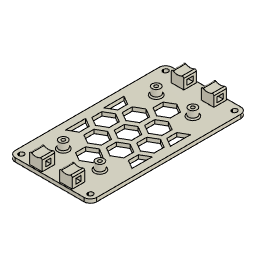
Lower Bay Tray - BIGTREETECH Relay 1.2 (Autodesk Fusion 360 design; units mm, degrees)
Autodesk Fusion 360 part; units mm, degrees
sketch "Base Sketch" plane through (0, 0, 0) normal (0, 0, 1) x (1, 0, 0)
  line L0 (-65, 70) -> (-10, 70) construction
  line L1 (-10, 70) -> (-10, 20) construction
  line L2 (-10, 20) -> (-65, 20) construction
  line L3 (-65, 20) -> (-65, 70) construction
  line L4 (-70, 20) -> (-70, 70)
  arc A0 (-65, 75) -> (-70, 70) centre (-65, 70) ccw
  arc A1 (-5, 70) -> (-10, 75) centre (-10, 70) ccw
  line L5 (-5, 70) -> (-5, 20)
  line L6 (-65, 75) -> (-10, 75)
  arc A2 (-70, 20) -> (-65, 15) centre (-65, 20) ccw
  line L7 (-10, 15) -> (-65, 15)
  arc A3 (-10, 15) -> (-5, 20) centre (-10, 20) ccw
  line L8 (-66.8, 70.25) -> (-66.8, 69.75)
  arc A4 (-66.8, 69.75) -> (-63.2, 69.75) centre (-65, 69.75) ccw
  line L9 (-63.2, 69.75) -> (-63.2, 70.25)
  arc A5 (-63.2, 70.25) -> (-66.8, 70.25) centre (-65, 70.25) ccw
  line L10 (-65, 70.25) -> (-65, 69.75) construction
  line L11 (-37.5, 75) -> (-37.5, 15) construction
  line L12 (-70, 45) -> (-5, 45) construction
  arc A6 (-66.8, 19.75) -> (-63.2, 19.75) centre (-65, 19.75) ccw
  line L13 (-66.8, 19.75) -> (-66.8, 20.25)
  arc A7 (-63.2, 20.25) -> (-66.8, 20.25) centre (-65, 20.25) ccw
  line L14 (-63.2, 20.25) -> (-63.2, 19.75)
  arc A8 (-8.2, 70.25) -> (-11.8, 70.25) centre (-10, 70.25) ccw
  line L15 (-8.2, 70.25) -> (-8.2, 69.75)
  arc A9 (-11.8, 69.75) -> (-8.2, 69.75) centre (-10, 69.75) ccw
  line L16 (-11.8, 69.75) -> (-11.8, 70.25)
  line L17 (-11.8, 20.25) -> (-11.8, 19.75)
  arc A10 (-8.2, 20.25) -> (-11.8, 20.25) centre (-10, 20.25) ccw
  line L18 (-8.2, 19.75) -> (-8.2, 20.25)
  arc A11 (-11.8, 19.75) -> (-8.2, 19.75) centre (-10, 19.75) ccw
  line L19 (70, 140) -> (70, 15) construction
  line L20 (70, 15) -> (5, 15) construction
  line L21 (5, 140) -> (70, 140) construction
  line L22 (5, 15) -> (5, 140) construction
  line L23 (10, 135) -> (65, 135) construction
  line L24 (65, 135) -> (65, 20) construction
  line L25 (65, 20) -> (10, 20) construction
  line L26 (10, 20) -> (10, 135) construction
  line L27 (65, 15) -> (10, 15)
  line L28 (5, 20) -> (5, 135)
  line L29 (10, 140) -> (65, 140)
  line L30 (70, 135) -> (70, 20)
  arc A12 (10, 140) -> (5, 135) centre (10, 135) ccw
  arc A13 (70, 135) -> (65, 140) centre (65, 135) ccw
  arc A14 (5, 20) -> (10, 15) centre (10, 20) ccw
  arc A15 (65, 15) -> (70, 20) centre (65, 20) ccw
  line L31 (8.1, 135.25) -> (8.1, 134.75)
  arc A16 (8.1, 134.75) -> (11.9, 134.75) centre (10, 134.75) ccw
  line L32 (11.9, 134.75) -> (11.9, 135.25)
  arc A17 (11.9, 135.25) -> (8.1, 135.25) centre (10, 135.25) ccw
  line L33 (10, 135.25) -> (10, 134.75) construction
  line L34 (37.5, 140) -> (37.5, 15) construction
  line L35 (5, 77.5) -> (70, 77.5) construction
  arc A18 (63.1, 134.75) -> (66.9, 134.75) centre (65, 134.75) ccw
  line L36 (63.1, 134.75) -> (63.1, 135.25)
  arc A19 (66.9, 135.25) -> (63.1, 135.25) centre (65, 135.25) ccw
  line L37 (66.9, 135.25) -> (66.9, 134.75)
  line L38 (66.9, 19.75) -> (66.9, 20.25)
  arc A20 (63.1, 19.75) -> (66.9, 19.75) centre (65, 19.75) ccw
  line L39 (63.1, 20.25) -> (63.1, 19.75)
  arc A21 (66.9, 20.25) -> (63.1, 20.25) centre (65, 20.25) ccw
  arc A22 (8.1, 19.75) -> (11.9, 19.75) centre (10, 19.75) ccw
  line L40 (8.1, 19.75) -> (8.1, 20.25)
  line L41 (11.9, 20.25) -> (11.9, 19.75)
  arc A23 (11.9, 20.25) -> (8.1, 20.25) centre (10, 20.25) ccw
  point P0 (-65, 70)
  point P1 (10, 135)
  point P2 (65, 135)
  point P3 (10, 20)
  point P4 (65, 20)
  point P5 (10, 135)
  dimension "d1" = 3.6
  dimension "d5" = 3.8
  constraint tangent L8 A4
  constraint tangent A4 L9
  constraint parallel L8 L9
  constraint tangent L9 A5
  constraint tangent L8 A5
  constraint vertical L10
  constraint coincident P0 L0.start
  constraint midpoint L10 P0
  constraint midpoint L6 L11.start
  constraint midpoint L7 L11.end
  constraint midpoint L4 L12.start
  constraint midpoint L5 L12.end
  constraint symmetric L8.start L12 A6.start
  constraint symmetric L8.end L12 L13.end
  constraint symmetric A4.end L12 A7.start
  constraint symmetric L9.end L12 A6.end
  constraint symmetric A4 L12 A7
  constraint symmetric A5 L12 A6
  constraint symmetric L8.start L11 A8.start
  constraint symmetric L8.end L11 L15.end
  constraint symmetric A4.end L11 A9.start
  constraint symmetric L9.end L11 A8.end
  constraint symmetric A4 L11 A9
  constraint symmetric A5 L11 A8
  constraint symmetric L11 A6.end L17.end
  constraint symmetric L11 A6.start L18.start
  constraint symmetric L11 A6 A11
  constraint symmetric L11 L13.end A10.start
  constraint symmetric L11 A7.start L17.start
  constraint symmetric L11 A7 A10
  constraint horizontal L23
  constraint vertical L24
  constraint horizontal L25
  constraint vertical L26
  constraint coincident P4 L24.end
  constraint coincident P5 P1
  constraint coincident L21 L29.start
  constraint parallel L25 L27
  constraint parallel L26 L28
  constraint parallel L23 L29
  constraint parallel L24 L30
  constraint coincident L21 L29.end
  constraint coincident P2 L23.end
  constraint coincident L22 L28.start
  constraint coincident P3 L25.end
  constraint tangent L31 A16
  constraint tangent A16 L32
  constraint parallel L31 L32
  constraint tangent L32 A17
  constraint tangent L31 A17
  constraint vertical L33
  constraint midpoint L33 P5
  constraint midpoint L21 L34.start
  constraint midpoint L20 L34.end
  constraint midpoint L28 L35.start
  constraint midpoint L19 L35.end
  constraint symmetric L31.start L34 A19.start
  constraint symmetric L31.end L34 A18.end
  constraint symmetric A16.end L34 A18.start
  constraint symmetric L32.end L34 L36.end
  constraint symmetric A16 L34 A18
  constraint symmetric A17 L34 A19
  constraint symmetric L31.start L35 A22.start
  constraint symmetric L31.end L35 L40.end
  constraint symmetric A16.end L35 L41.start
  constraint symmetric L32.end L35 A22.end
  constraint symmetric A16 L35 A23
  constraint symmetric A17 L35 A22
  constraint symmetric L35 A18.end L38.end
  constraint symmetric L35 A18.start L39.start
  constraint symmetric L35 A18 A21
  constraint symmetric L35 L36.end A20.start
  constraint symmetric L35 A19.start L38.start
  constraint symmetric L35 A19 A20
  measures "d1" diameter of A4
  measures "d5" diameter of A16
extrude "Extrude1" add sketch "Base Sketch" along normal blind 3 contours L27 L28 L29 L30 A12 A13 A14 A15 makes body 1 in component "Dual Buck"
ref_plane "WorkPlane1" through (0, 0, 3) normal (0, 0, 1) x (1, 0, 0)
copy_body "CopyPasteBodies1" bodies 1 makes body 2 in component "Single Buck"
move_body "Move1" bodies 2 to x (1, 0, 0) y (0, 1, 0) z (0, 0, 1) at (-75, 0, 0) in component "Single Buck"
sketch "Single Buck" plane through (0, 0, 3) normal (0, 0, 1) x (-1, 0, 0)
  arc A0 (8.1, -20.25) -> (11.9, -20.25) centre (10, -20.25) ccw
  line L0 (8.1, -20.25) -> (8.1, -19.75)
  arc A1 (11.9, -19.75) -> (8.1, -19.75) centre (10, -19.75) ccw
  line L1 (11.9, -19.75) -> (11.9, -20.25)
  arc A2 (63.1, -135.25) -> (66.9, -135.25) centre (65, -135.25) ccw
  line L2 (63.1, -135.25) -> (63.1, -134.75)
  arc A3 (66.9, -134.75) -> (63.1, -134.75) centre (65, -134.75) ccw
  line L3 (66.9, -134.75) -> (66.9, -135.25)
  arc A4 (66.9, -19.75) -> (63.1, -19.75) centre (65, -19.75) ccw
  line L4 (66.9, -19.75) -> (66.9, -20.25)
  arc A5 (63.1, -20.25) -> (66.9, -20.25) centre (65, -20.25) ccw
  line L5 (63.1, -20.25) -> (63.1, -19.75)
  arc A6 (11.9, -134.75) -> (8.1, -134.75) centre (10, -134.75) ccw
  line L6 (11.9, -134.75) -> (11.9, -135.25)
  arc A7 (8.1, -135.25) -> (11.9, -135.25) centre (10, -135.25) ccw
  line L7 (8.1, -135.25) -> (8.1, -134.75)
  arc A8 (70, -20) -> (65, -15) centre (65, -20) ccw
  line L8 (65, -15) -> (10, -15)
  arc A9 (10, -15) -> (5, -20) centre (10, -20) ccw
  line L9 (5, -20) -> (5, -135)
  arc A10 (5, -135) -> (10, -140) centre (10, -135) ccw
  line L10 (10, -140) -> (65, -140)
  arc A11 (65, -140) -> (70, -135) centre (65, -135) ccw
  line L11 (70, -135) -> (70, -20)
  line L12 (22.895, -40.464) -> (52.105, -40.464) construction
  line L13 (52.105, -40.464) -> (52.105, -114.634) construction
  line L14 (52.105, -114.634) -> (22.895, -114.634) construction
  line L15 (22.895, -114.634) -> (22.895, -40.464) construction
  circle A12 centre (22.895, -114.634) radius 1.4
  circle A13 centre (22.895, -40.464) radius 1.4
  circle A14 centre (52.105, -40.464) radius 1.4
  circle A15 centre (52.105, -114.634) radius 1.4
  circle A16 centre (52.105, -114.634) radius 3.5
  circle A17 centre (22.895, -114.634) radius 3.5
  circle A18 centre (22.895, -40.464) radius 3.5
  circle A19 centre (52.105, -40.464) radius 3.5
  line L16 (70, -77.5) -> (5, -77.5) construction
  line L17 (37.5, -140) -> (37.5, -15) construction
  point P0 (52.105, -77.549)
  point P1 (37.5, -114.634)
  dimension "d38" = 7
  dimension "d39" = 7
  dimension "d40" = 7
  dimension "d41" = 7
  dimension "d75" = 29.21
  dimension "d76" = 74.17
  dimension "d79" = 2.8
  dimension "d80" = 2.8
  dimension "d81" = 2.8
  dimension "d82" = 2.8
  constraint coincident L13.end L14.start
  constraint coincident L14.end L15.start
  constraint coincident L12.start L15.end
  constraint coincident L12.end L13.start
  constraint midpoint L11 L16.start
  constraint midpoint L9 L16.end
  constraint midpoint L13 P0
  constraint horizontal L14
  constraint vertical L15
  constraint horizontal L12
  constraint vertical L13
  constraint midpoint L10 L17.start
  constraint midpoint L8 L17.end
  constraint midpoint L14 P1
  constraint coincident L17 P1
  measures "d38" diameter of A16
  measures "d39" diameter of A17
  measures "d40" diameter of A18
  measures "d41" diameter of A19
  measures "d75" distance of L13.end L14.end
  measures "d76" distance of L12.end L13.end
  measures "d79" diameter of A14
  measures "d80" diameter of A15
  measures "d81" diameter of A12
  measures "d82" diameter of A13
extrude "Extrude1'" add sketch "Single Buck" along normal blind 6 draft -1.5 contours A12 | A13 | A14 | A15 | A16 | A17 | A18 | A19 bodies 2 in component "Single Buck"
extrude "Extrude8" cut sketch "Single Buck" against normal blind 13 from surface at 6 contours A12 | A13 | A14 | A15 bodies 2 in component "Single Buck"
fillet "Fillet1" radius 1 4 edges at (-48.8419, 39.1984, 3) (-48.8419, 113.3684, 3) (-19.6319, 113.3684, 3) (-19.6319, 39.1984, 3) on bodies 2 in component "Single Buck"
ref_plane "WorkPlane2" through (0, 15, 0) normal (0, 1, 0) x (0, 0, 1)
sketch "Wire Anchors" plane through (0, 15, 0) normal (0, 1, 0) x (1, 0, 0)
  line L0 (-65, -3) -> (-10, -3)
  line L1 (-44.5, -3) -> (-54.5, -3)
  line L2 (-54.5, -3) -> (-54.5, -11.0007)
  line L3 (-44.5, -11.0007) -> (-44.5, -3)
  arc A0 (-46, -11.8668) -> (-53, -11.8668) centre (-49.5, -17.9289) ccw
  arc A1 (-54.5, -11.0007) -> (-53, -11.8668) centre (-53.5, -11.0007) ccw
  arc A2 (-46, -11.8668) -> (-44.5, -11.0007) centre (-45.5, -11.0007) ccw
  arc A3 (-44.5, -9) -> (-54.5, -9) centre (-49.5, -17.0333) ccw
  line L4 (-53, -11.8668) -> (-46, -11.8668) construction
  line L5 (-53.5, -11.0007) -> (-45.5, -11.0007) construction
  line L6 (-54.5, -9) -> (-44.5, -9) construction
  line L7 (-44.5, -5) -> (-54.5, -5)
  line L8 (-37.5, -3) -> (-37.5, -19.5188) construction
  line L9 (-20.5, -3) -> (-20.5, -11.0007)
  arc A4 (-22, -11.8668) -> (-20.5, -11.0007) centre (-21.5, -11.0007) ccw
  arc A5 (-22, -11.8668) -> (-29, -11.8668) centre (-25.5, -17.9289) ccw
  arc A6 (-30.5, -11.0007) -> (-29, -11.8668) centre (-29.5, -11.0007) ccw
  line L10 (-30.5, -11.0007) -> (-30.5, -3)
  line L11 (-30.5, -3) -> (-20.5, -3)
  arc A7 (-20.5, -9) -> (-30.5, -9) centre (-25.5, -17.0333) ccw
  line L12 (-30.5, -5) -> (-20.5, -5)
  point P0 (-31.5, -8)
  dimension "d49" = 1
  dimension "d50" = 1
  dimension "d91" = 10
  dimension "d95" = 6
  dimension "d96" = -2
  constraint horizontal L1
  constraint perpendicular L1 L2
  constraint parallel L2 L3
  constraint tangent L2 A1
  constraint tangent A0 A1
  constraint tangent A0 A2
  constraint tangent L3 A2
  constraint coincident L3 A3.start
  constraint coincident L2 A3.end
  constraint collinear L0 L1
  constraint coincident A1.centre L5.start
  constraint coincident A2.centre L5.end
  constraint perpendicular L3 L6
  constraint midpoint L0 L8.start
  constraint perpendicular L0 L8
  constraint symmetric L1.start L8 L10.end
  constraint symmetric L1.end L8 L9.start
  constraint symmetric A0 L8 A5
  constraint symmetric L2.end L8 L9.end
  constraint symmetric A0.end L8 A4.start
  constraint symmetric A1 L8 A4
  constraint symmetric L3.start L8 A6.start
  constraint symmetric A0.start L8 A5.end
  constraint symmetric A2 L8 A6
  constraint symmetric A3.start L8 A7.end
  constraint symmetric A3.end L8 A7.start
  constraint symmetric A3 L8 A7
  constraint symmetric L7.start L8 L12.start
  constraint symmetric L7.end L8 L12.end
  measures "d49" radius of A1
  measures "d50" radius of A2
  measures "d91" distance of L2 L3
  measures "d95" distance of L1.end A3.end
extrude "Extrude2" add sketch "Wire Anchors" along normal blind 10 from surface at 1 bodies 2 in component "Single Buck"
extrude "Extrude3" add sketch "Wire Anchors" against normal blind 10 from surface at 124 bodies 2 in component "Single Buck"
extrude "Extrude4" cut sketch "Wire Anchors" along normal mid plane 4 from surface at 6 contours L2 L3 A3 L7 | L9 L10 A7 L12 bodies 2 in component "Single Buck"
extrude "Extrude5" cut sketch "Wire Anchors" along normal blind 5 and the other way blind 0 from surface at 116.5 contours L2 L3 A3 L7 | L9 L10 A7 L12 bodies 2 in component "Single Buck"
sketch "Sketch5" plane through (0, 0, 3) normal (0, 0, 1) x (-1, 0, 0)
  line L0 (20.5, -129) -> (30.5, -129)
  line L1 (30.5, -26) -> (20.5, -26)
  arc A0 (70, -20) -> (65, -15) centre (65, -20) ccw
  line L2 (65, -15) -> (10, -15)
  arc A1 (10, -15) -> (5, -20) centre (10, -20) ccw
  line L3 (5, -20) -> (5, -135)
  arc A2 (5, -135) -> (10, -140) centre (10, -135) ccw
  line L4 (10, -140) -> (65, -140)
  arc A3 (65, -140) -> (70, -135) centre (65, -135) ccw
  line L5 (70, -135) -> (70, -20)
  arc A4 (11.9, -134.75) -> (8.1, -134.75) centre (10, -134.75) ccw
  line L6 (11.9, -134.75) -> (11.9, -135.25)
  arc A5 (8.1, -135.25) -> (11.9, -135.25) centre (10, -135.25) ccw
  line L7 (8.1, -135.25) -> (8.1, -134.75)
  arc A6 (66.9, -19.75) -> (63.1, -19.75) centre (65, -19.75) ccw
  line L8 (66.9, -19.75) -> (66.9, -20.25)
  arc A7 (63.1, -20.25) -> (66.9, -20.25) centre (65, -20.25) ccw
  line L9 (63.1, -20.25) -> (63.1, -19.75)
  arc A8 (63.1, -135.25) -> (66.9, -135.25) centre (65, -135.25) ccw
  line L10 (63.1, -135.25) -> (63.1, -134.75)
  arc A9 (66.9, -134.75) -> (63.1, -134.75) centre (65, -134.75) ccw
  line L11 (66.9, -134.75) -> (66.9, -135.25)
  arc A10 (8.1, -20.25) -> (11.9, -20.25) centre (10, -20.25) ccw
  line L12 (8.1, -20.25) -> (8.1, -19.75)
  arc A11 (11.9, -19.75) -> (8.1, -19.75) centre (10, -19.75) ccw
  line L13 (11.9, -19.75) -> (11.9, -20.25)
  line L14 (37.5, -15) -> (37.5, -140) construction
  line L15 (70, -77.5) -> (5, -77.5) construction
  line L16 (37.5, -85.5) -> (44.4282, -81.5)
  line L17 (44.4282, -81.5) -> (44.4282, -73.5)
  line L18 (44.4282, -73.5) -> (37.5, -69.5)
  line L19 (37.5, -69.5) -> (30.5718, -73.5)
  line L20 (30.5718, -73.5) -> (30.5718, -81.5)
  line L21 (30.5718, -81.5) -> (37.5, -85.5)
  line L22 (62.1962, -81.366) -> (62.1962, -73.366)
  line L23 (62.1962, -73.366) -> (55.268, -69.366)
  line L24 (55.268, -69.366) -> (48.3397, -73.366)
  line L25 (48.3397, -73.366) -> (48.3397, -81.366)
  line L26 (48.3397, -81.366) -> (55.2679, -85.366)
  line L27 (55.2679, -85.366) -> (62.1962, -81.366)
  line L28 (53.1962, -58.0455) -> (46.268, -54.0455)
  line L29 (46.268, -54.0455) -> (39.3397, -58.0455)
  line L30 (39.3397, -58.0455) -> (39.3397, -66.0455)
  line L31 (39.3397, -66.0455) -> (46.2679, -70.0455)
  line L32 (46.2679, -70.0455) -> (53.1962, -66.0455)
  line L33 (53.1962, -66.0455) -> (53.1962, -58.0455)
  line L34 (28.5, -54.1795) -> (21.5718, -58.1795)
  line L35 (21.5718, -58.1795) -> (21.5718, -66.1795)
  line L36 (21.5718, -66.1795) -> (28.5, -70.1795)
  line L37 (28.5, -70.1795) -> (35.4282, -66.1795)
  line L38 (35.4282, -66.1795) -> (35.4282, -58.1795)
  line L39 (35.4282, -58.1795) -> (28.5, -54.1795)
  line L40 (12.8038, -73.634) -> (12.8038, -81.634)
  line L41 (12.8038, -81.634) -> (19.7321, -85.634)
  line L42 (19.7321, -85.634) -> (26.6603, -81.634)
  line L43 (26.6603, -81.634) -> (26.6603, -73.634)
  line L44 (26.6603, -73.634) -> (19.7321, -69.634)
  line L45 (19.7321, -69.634) -> (12.8038, -73.634)
  line L46 (21.8038, -96.9545) -> (28.7321, -100.9545)
  line L47 (28.7321, -100.9545) -> (35.6603, -96.9545)
  line L48 (35.6603, -96.9545) -> (35.6603, -88.9545)
  line L49 (35.6603, -88.9545) -> (28.7321, -84.9545)
  line L50 (28.7321, -84.9545) -> (21.8038, -88.9545)
  line L51 (21.8038, -88.9545) -> (21.8038, -96.9545)
  line L52 (46.5, -100.8205) -> (53.4282, -96.8205)
  line L53 (53.4282, -96.8205) -> (53.4282, -88.8205)
  line L54 (53.4282, -88.8205) -> (46.5, -84.8205)
  line L55 (46.5, -84.8205) -> (39.5718, -88.8205)
  line L56 (39.5718, -88.8205) -> (39.5718, -96.8205)
  line L57 (39.5718, -96.8205) -> (46.5, -100.8205)
  circle A12 centre (52.105, -40.464) radius 4.4742
  circle A13 centre (22.895, -40.464) radius 4.4742
  line L58 (54.5, -129) -> (54.5, -139)
  line L59 (30.5, -139) -> (20.5, -139)
  line L60 (44.5, -139) -> (44.5, -129)
  line L61 (44.5, -26) -> (44.5, -16)
  line L62 (20.5, -16) -> (30.5, -16)
  line L63 (54.5, -16) -> (54.5, -26)
  circle A14 centre (22.895, -114.634) radius 4.4742
  circle A15 centre (52.105, -114.634) radius 4.4742
  line L64 (20.5, -26) -> (20.5, -16)
  line L65 (30.5, -16) -> (30.5, -26)
  line L66 (54.5, -26) -> (44.5, -26)
  line L67 (30.5, -129) -> (30.5, -139)
  line L68 (20.5, -139) -> (20.5, -129)
  line L69 (44.5, -129) -> (54.5, -129)
  line L70 (54.5, -139) -> (44.5, -139)
  line L71 (44.5, -16) -> (54.5, -16)
  line L72 (46.5, -84.8205) -> (46.5, -100.8205) construction
  line L73 (55.2679, -85.366) -> (55.2679, -94.9794) construction
  line L74 (64.0359, -100.8205) -> (57.1077, -96.8205)
  line L75 (57.1077, -96.8205) -> (57.1077, -88.8205)
  line L76 (57.1077, -88.8205) -> (64.0359, -84.8205)
  line L77 (64.0359, -100.8205) -> (64.0359, -84.8205)
  line L78 (17.8923, -88.8205) -> (10.9641, -84.8205)
  line L79 (17.8923, -96.8205) -> (17.8923, -88.8205)
  line L80 (10.9641, -100.8205) -> (17.8923, -96.8205)
  line L81 (10.9641, -100.8205) -> (10.9641, -84.8205)
  line L82 (17.8923, -66.1795) -> (10.9641, -70.1795)
  line L83 (10.9641, -54.1795) -> (10.9641, -70.1795)
  line L84 (10.9641, -54.1795) -> (17.8923, -58.1795)
  line L85 (17.8923, -58.1795) -> (17.8923, -66.1795)
  line L86 (57.1077, -66.1795) -> (64.0359, -70.1795)
  line L87 (64.0359, -54.1795) -> (64.0359, -70.1795)
  line L88 (57.1077, -58.1795) -> (57.1077, -66.1795)
  line L89 (64.0359, -54.1795) -> (57.1077, -58.1795)
  line L90 (35.6603, -92.9545) -> (29.3092, -92.9545) construction
  line L91 (44.4282, -104.409) -> (44.4282, -112.409)
  line L92 (44.4282, -112.409) -> (37.5, -116.409)
  line L93 (37.5, -116.409) -> (30.5718, -112.409)
  line L94 (30.5718, -112.409) -> (30.5718, -104.409)
  line L95 (30.5718, -104.409) -> (37.5, -100.409)
  line L96 (37.5, -100.409) -> (44.4282, -104.409)
  line L97 (44.4282, -50.591) -> (44.4282, -42.591)
  line L98 (44.4282, -42.591) -> (37.5, -38.591)
  line L99 (37.5, -38.591) -> (30.5718, -42.591)
  line L100 (30.5718, -42.591) -> (30.5718, -50.591)
  line L101 (30.5718, -50.591) -> (37.5, -54.591)
  line L102 (37.5, -54.591) -> (44.4282, -50.591)
  point P0 (37.5, -77.5)
  dimension "d86" = 8
  dimension "d88" = 360
  constraint midpoint L2 L14.start
  constraint midpoint L4 L14.end
  constraint midpoint L5 L15.start
  constraint midpoint L3 L15.end
  constraint midpoint L15 P0
  constraint vertical L72
  constraint vertical L56
  constraint vertical L53
  constraint symmetric L53 L56 L72
  constraint symmetric L52 L57 L72
  constraint symmetric L54 L55 L72
  constraint parallel L72 L73
  constraint symmetric L52.start L73 L74.start
  constraint symmetric L52.end L73 L74.end
  constraint symmetric L53.end L73 L75.end
  constraint symmetric L54.end L73 L76.end
  constraint symmetric L14 L74.start L80.start
  constraint symmetric L14 L74.end L79.start
  constraint symmetric L14 L75.end L78.start
  constraint symmetric L14 L76.end L78.end
  constraint symmetric L15 L74.start L87.start
  constraint symmetric L15 L74.end L88.start
  constraint symmetric L15 L75.end L86.start
  constraint symmetric L15 L76.end L86.end
  constraint symmetric L15 L78.start L82.start
  constraint symmetric L15 L78.end L82.end
  constraint symmetric L15 L79.start L84.end
  constraint symmetric L15 L80.start L83.start
  constraint midpoint L48 L90.start
  constraint perpendicular L48 L90
  constraint symmetric L16.start L90 L95.end
  constraint symmetric L16.end L90 L91.start
  constraint symmetric L17.end L90 L91.end
  constraint symmetric L18.end L90 L92.end
  constraint symmetric L19.end L90 L93.end
  constraint symmetric L20.end L90 L94.end
  constraint symmetric L15 L91.start L97.start
  constraint symmetric L15 L91.end L97.end
  constraint symmetric L15 L92.end L98.end
  constraint symmetric L15 L93.end L99.end
  constraint symmetric L15 L94.end L100.end
  constraint symmetric L15 L95.end L101.end
  measures "d86" distance of L16.start P0
extrude "Extrude9" cut sketch "Sketch5" against normal blind 3 contours L16 L17 L18 L19 L20 L21 | L22 L23 L24 L25 L26 L27 | L28 L29 L30 L31 L32 L33 | L34 L35 L36 L37 L38 L39 | L40 L41 L42 L43 L44 L45 | L46 L47 L48 L49 L50 L51 | L52 L53 L54 L55 L56 L57 | L74 L75 L76 L77 | L78 L79 L80 L81 | L82 L83 L84 L85 | L86 L87 L88 L89 | L91 L92 L93 L94 L95 L96 | L97 L98 L99 L100 L101 L102 bodies 2 in component "Single Buck"
component "Single Buck" placed x (1, 0, 0) y (0, 1, 0) z (0, 0, 1) at (0, 0, 0)
equation "short_len = 40.5 mm" comment "Shorter side of the mounting hole rect"
equation "long_len = 63 mm" comment "Larger side of the mounting hole rect"
equation "hole_dia = 2.8 mm" comment "Mounting hole diameter"
equation "d39 = d38"
equation "d40 = d38"
equation "d41 = d38"
